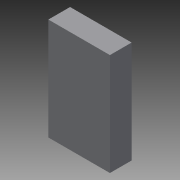
# Autodesk Inventor part: dlink5portswitch
Saved by Autodesk Inventor 2015 (Build 190159000, 159)
## iProperties
Created: 2014-09-28
Part Number: dlink5portswitch
Material: Generic
Document SubType Name: Modeling
Designer: ericd_000
Density: 1 g/cm^3
Appearance: Default
Author: ericd_000
Autodesk Inventor part; units mm, degrees
ref_plane "YZ Plane" through (0, 0, 0) normal (1, 0, 0) x (0, 1, 0)
ref_plane "XZ Plane" through (0, 0, 0) normal (0, 1, 0) x (-1, 0, 0)
ref_plane "XY Plane" through (0, 0, 0) normal (0, 0, 1) x (1, 0, 0)
sketch "Sketch1" plane through (0, 0, 0) normal (0, 1, 0) x (-1, 0, 0)
  line L0 (42.5, 70.5) -> (-42.5, 70.5)
  line L1 (-42.5, 70.5) -> (-42.5, -70.5)
  line L2 (-42.5, -70.5) -> (42.5, -70.5)
  line L3 (42.5, -70.5) -> (42.5, 70.5)
  point P0 (0, 0)
  point P1 (42.5, 0)
  point P2 (0, 70.5)
  dimension "d0" = 141
  dimension "d1" = 85
  constraints: 8 end point, 2 midpoint, 2 parallel, 1 horizontal, 1 horizontal alignment, 1 perpendicular, 1 vertical alignment
  measures "d0" distance of L2.end L0.start
  measures "d1" distance of L0.start L0.end
extrude "Extrusion1" add sketch "Sketch1" along normal blind 30
body "Solid1"
